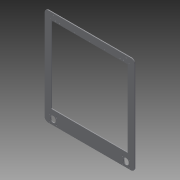
# Autodesk Inventor part: 300 mm top plate
Saved by Autodesk Inventor 2014 SP1 (Build 180222100, 222)
## iProperties
Created: 2014-10-03
Part Number: 300 mm top plate
Material: Generic
Document SubType Name: Modeling
Designer: Mon
Density: 1 g/cm^3
Appearance: Default
Author: Mon
Autodesk Inventor part; units mm, degrees
ref_plane "YZ Plane" through (0, 0, 0) normal (1, 0, 0) x (0, 1, 0)
ref_plane "XZ Plane" through (0, 0, 0) normal (0, 1, 0) x (-1, 0, 0)
ref_plane "XY Plane" through (0, 0, 0) normal (0, 0, 1) x (1, 0, 0)
sketch "Sketch2" plane through (0, 0, 0) normal (0, 1, 0) x (-1, 0, 0)
  line L0 (381.1115, 61.7853) -> (30.3977, 61.7853)
  line L1 (380.9072, 412.5623) -> (381.1115, 61.7853)
  line L2 (30.1934, 412.5623) -> (380.9072, 412.5623)
  line L3 (30.3977, 61.7853) -> (30.3977, 412.5623)
  arc A0 (0.0977, 16.0853) -> (16.0601, 0.0853) centre (16.0335, 16.0213) ccw
  line L4 (0.0977, 16.0853) -> (-0.1066, 429.5623)
  arc A1 (15.8934, 445.5623) -> (-0.1066, 429.5623) centre (15.8934, 429.5623) ccw
  line L5 (15.8934, 445.5623) -> (395.2072, 445.5623)
  arc A2 (411.2072, 429.5623) -> (395.2072, 445.5623) centre (395.2072, 429.5623) ccw
  line L6 (411.2072, 429.5623) -> (411.4115, 16.0853)
  arc A3 (395.3739, 0.0853) -> (411.4115, 16.0853) centre (395.3472, 16.1497) ccw
  line L7 (395.3739, 0.0853) -> (16.0601, 0.0853)
  arc A4 (21.3351, 6.5853) -> (25.0851, 6.5853) centre (23.2101, 6.5853) ccw
  line L8 (25.0851, 10.5853) -> (25.0851, 6.5853)
  arc A5 (25.0851, 10.5853) -> (21.3351, 10.5853) centre (23.2101, 10.5853) ccw
  line L9 (21.3351, 6.5853) -> (21.3351, 10.5853)
  arc A6 (52.3351, 6.5853) -> (56.0851, 6.5853) centre (54.2101, 6.5853) ccw
  line L10 (56.0851, 10.5853) -> (56.0851, 6.5853)
  arc A7 (56.0851, 10.5853) -> (52.3351, 10.5853) centre (54.2101, 10.5853) ccw
  line L11 (52.3351, 6.5853) -> (52.3351, 10.5853)
  arc A8 (21.3351, 37.5853) -> (25.0851, 37.5853) centre (23.2101, 37.5853) ccw
  line L12 (25.0851, 41.5853) -> (25.0851, 37.5853)
  arc A9 (25.0851, 41.5853) -> (21.3351, 41.5853) centre (23.2101, 41.5853) ccw
  line L13 (21.3351, 37.5853) -> (21.3351, 41.5853)
  arc A10 (52.3351, 37.5853) -> (56.0851, 37.5853) centre (54.2101, 37.5853) ccw
  line L14 (56.0851, 41.5853) -> (56.0851, 37.5853)
  arc A11 (56.0851, 41.5853) -> (52.3351, 41.5853) centre (54.2101, 41.5853) ccw
  line L15 (52.3351, 37.5853) -> (52.3351, 41.5853)
  arc A12 (26.7101, 22.0853) -> (50.7101, 22.0853) centre (38.7101, 22.0853) ccw
  line L16 (50.7101, 26.0853) -> (50.7101, 22.0853)
  arc A13 (50.7101, 26.0853) -> (26.7101, 26.0853) centre (38.7101, 26.0853) ccw
  line L17 (26.7101, 22.0853) -> (26.7101, 26.0853)
  arc A14 (355.3489, 6.5853) -> (359.1299, 6.5853) centre (357.2394, 6.6008) ccw
  line L18 (359.1299, 10.5853) -> (359.1299, 6.5853)
  arc A15 (359.1299, 10.5853) -> (355.3489, 10.5853) centre (357.2394, 10.5698) ccw
  line L19 (355.3489, 6.5853) -> (355.3489, 10.5853)
  arc A16 (386.3313, 6.5853) -> (390.0989, 6.577) centre (388.215, 6.5376) ccw
  arc A17 (386.3384, 37.5853) -> (390.0884, 37.5853) centre (388.2134, 37.5853) ccw
  line L20 (390.0884, 41.5853) -> (390.0884, 37.5853)
  arc A18 (390.0884, 41.5853) -> (386.3384, 41.5853) centre (388.2134, 41.5853) ccw
  line L21 (386.3384, 37.5853) -> (386.3384, 41.5853)
  arc A19 (355.3298, 37.5853) -> (359.0798, 37.5853) centre (357.2048, 37.5853) ccw
  line L22 (359.0798, 41.5853) -> (359.0798, 37.5853)
  arc A20 (359.0798, 41.5853) -> (355.3489, 41.5853) centre (357.2143, 41.5948) ccw
  line L23 (355.3298, 37.5853) -> (355.3489, 41.5853)
  arc A21 (360.6847, 22.0853) -> (384.6847, 22.0853) centre (372.6847, 22.0853) ccw
  line L24 (384.6847, 26.0853) -> (384.6847, 22.0853)
  arc A22 (384.6847, 26.0853) -> (360.6847, 26.0853) centre (372.6847, 26.0853) ccw
  line L25 (360.6847, 22.0853) -> (360.6847, 26.0853)
  circle A23 centre (50.1434, 420.5623) radius 2.1
  circle A24 centre (38.5434, 435.5623) radius 2.1
  circle A25 centre (372.5572, 435.5623) radius 2.1
  circle A26 centre (360.9572, 420.5623) radius 2.1
  circle A27 centre (25.7809, 418.0623) radius 1.6
  circle A28 centre (66.7809, 418.0623) radius 1.6
  circle A29 centre (205.5503, 418.0623) radius 1.6
  circle A30 centre (344.3197, 418.0623) radius 1.6
  circle A31 centre (386.2129, 418.0623) radius 1.6
  circle A32 centre (385.3197, 56.2853) radius 1
  circle A33 centre (344.3197, 56.2853) radius 1
  circle A34 centre (205.5503, 56.2853) radius 1
  circle A35 centre (66.7809, 56.2853) radius 1
  circle A36 centre (25.7809, 56.2853) radius 1
  arc A37 (390.0989, 10.5853) -> (386.3489, 10.5853) centre (388.2239, 10.5853) ccw
  line L26 (378.8199, 179.5488) -> (32.1952, 179.5488)
  circle A38 centre (60.6452, 222.8238) radius 1.6
  circle A39 centre (60.6452, 258.6363) radius 1.6
  circle A40 centre (60.6452, 187.0113) radius 1.6
  circle A41 centre (350.3699, 187.0113) radius 1.6
  circle A42 centre (350.3699, 222.8238) radius 1.6
  circle A43 centre (350.3699, 258.6363) radius 1.6
  circle A44 centre (49.8452, 185.8988) radius 1.6
  circle A45 centre (49.8452, 259.7488) radius 1.6
  circle A46 centre (361.1699, 222.8238) radius 1.6
  line L27 (378.8199, 266.0988) -> (378.8199, 179.5488)
  line L28 (345.8699, 256.5738) -> (345.8699, 189.0738)
  line L29 (65.1452, 256.5738) -> (345.8699, 256.5738)
  line L30 (65.1452, 189.0738) -> (65.1452, 256.5738)
  line L31 (345.8699, 189.0738) -> (65.1452, 189.0738)
  line L32 (32.1952, 179.5488) -> (32.1952, 266.0988)
  line L33 (32.1952, 266.0988) -> (378.8199, 266.0988)
  circle A47 centre (50.1452, 204.5238) radius 2.1
  circle A48 centre (360.8699, 204.5238) radius 2.1
  circle A49 centre (360.8699, 241.1238) radius 2.1
  circle A50 centre (50.1452, 241.1238) radius 2.1
  line L34 (224.6003, 203.7738) -> (186.5003, 203.7738)
  line L35 (224.6003, 207.8328) -> (224.6003, 203.7738)
  arc A51 (226.0103, 209.3301) -> (224.6003, 207.8328) centre (226.1003, 207.8328) ccw
  arc A52 (226.0103, 209.3301) -> (226.0103, 216.3175) centre (225.8003, 212.8238) ccw
  arc A53 (224.6003, 217.8148) -> (226.0103, 216.3175) centre (226.1003, 217.8148) ccw
  arc A54 (226.0103, 229.3301) -> (224.6003, 227.8328) centre (226.1003, 227.8328) ccw
  arc A55 (226.0103, 229.3301) -> (226.0103, 236.3175) centre (225.8003, 232.8238) ccw
  arc A56 (224.6003, 237.8148) -> (226.0103, 236.3175) centre (226.1003, 237.8148) ccw
  line L36 (186.5003, 241.8738) -> (224.6003, 241.8738)
  line L37 (186.5003, 237.8148) -> (186.5003, 241.8738)
  arc A57 (185.0903, 236.3175) -> (186.5003, 237.8148) centre (185.0003, 237.8148) ccw
  arc A58 (185.0903, 236.3175) -> (185.0903, 229.3301) centre (185.3003, 232.8238) ccw
  arc A59 (186.5003, 227.8328) -> (185.0903, 229.3301) centre (185.0003, 227.8328) ccw
  arc A60 (185.0903, 216.3175) -> (186.5003, 217.8148) centre (185.0003, 217.8148) ccw
  arc A61 (185.0903, 216.3175) -> (185.0903, 209.3301) centre (185.3003, 212.8238) ccw
  arc A62 (186.5003, 207.8328) -> (185.0903, 209.3301) centre (185.0003, 207.8328) ccw
  line L38 (173.8003, 254.5738) -> (237.3003, 254.5738)
  line L39 (237.3003, 254.5738) -> (237.3003, 191.0738)
  line L40 (237.3003, 191.0738) -> (173.8003, 191.0738)
  line L41 (173.8003, 191.0738) -> (173.8003, 254.5738)
  circle A63 centre (180.1503, 197.0113) radius 0.875
  circle A64 centre (230.9503, 197.0113) radius 0.875
  circle A65 centre (230.9503, 248.6363) radius 0.875
  circle A66 centre (180.1503, 248.6363) radius 0.875
  circle A67 centre (177.8003, 232.8238) radius 0.875
  circle A68 centre (233.3003, 232.8238) radius 0.875
  circle A69 centre (233.3003, 212.8238) radius 0.875
  circle A70 centre (177.8003, 212.8238) radius 0.875
  line L42 (186.5003, 203.7738) -> (186.5003, 207.8328)
  line L43 (186.5003, 217.8148) -> (186.5003, 227.8328)
  line L44 (224.6003, 241.8738) -> (224.6003, 237.8148)
  line L45 (224.6003, 227.8328) -> (224.6003, 217.8148)
  line L46 (390.0989, 10.5853) -> (390.0989, 6.577)
  line L47 (386.3489, 10.5853) -> (386.3313, 6.5853)
  circle A71 centre (136.7809, 56.2853) radius 1
  circle A72 centre (273.8132, 56.2853) radius 1
  circle A73 centre (274.3197, 418.0623) radius 1.6
  circle A74 centre (136.7809, 418.0623) radius 1.6
  point P0 (0, 0)
  constraints: 96 end point, 75 centre point, 72 point on circle, 1 point on line
extrude "Extrusion1" add sketch "Sketch2" along normal blind 4 contours L4 A1 L5 A2 L6 A3 L7 A0
body "Solid1"
